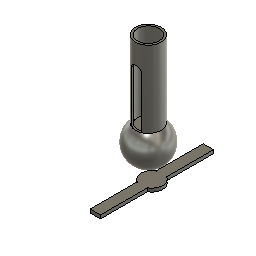
Tube and Handle (Autodesk Fusion 360 design; units mm, degrees)
part number: 2026-07-05-17-09-31-092
Autodesk Fusion 360 part; units mm, degrees
sphere "SpherePrimitive1" add diameter 80 placed x (1, 0, 0) y (0, 0, -1) z (0, 1, 0) at (0, 0, 0) makes body 1
sketch "Sketch2" plane through (0, 0, 0) normal (0, 1, 0) x (1, 0, 0)
  circle A0 centre (0, 0) radius 25
  dimension "d2" = 50
  constraint coincident A0.centre origin
  measures "d2" diameter of A0
extrude "Extrude1" add sketch "Sketch2" along normal blind 200 bodies 1
hole "Hole1" at (0, 200, 0) direction (0, -1, 0) diameter 42 depth 170 tip angle 180 bodies 1
extrude "Extrude2" cut 1 faces at (23.554, 200, 1.7651) along direction (0, -1, 0) blind 20 on bodies 1 bodies 1
sketch "Sketch3" plane through (0, 0, 0) normal (0, 0, 1) x (1, 0, 0)
  line L0 (-25, 31.225) -> (25, 31.225)
  line L1 (-25, 180) -> (25, 180)
  line L2 (10, 31.225) -> (-10, 31.225)
  line L3 (-10, 31.225) -> (-10, 131.225)
  line L4 (10, 131.225) -> (10, 31.225)
  arc A0 (0, 141.225) -> (-10, 131.225) centre (0, 131.225) ccw
  arc A1 (10, 131.225) -> (0, 141.225) centre (0, 131.225) ccw
  point P0 (10, 141.225)
  dimension "d10" = 20
  dimension "d11" = 110
  dimension "d12" = 15
  dimension "d13" = 10
  dimension "d14" = 10
  constraint horizontal L2
  constraint vertical L3
  constraint vertical L4
  constraint coincident L0 L2.start
  constraint tangent L3 A0
  constraint coincident P0 L4
  constraint tangent L4 A1
  constraint coincident A0.start A1.end
  measures "d10" distance of L2.start L2.end
  measures "d11" distance of L2.start P0
  measures "d12" distance of L0.end L4
  measures "d13" radius of A0
  measures "d14" radius of A1
extrude "Extrude3" cut sketch "Sketch3" along normal blind 30 and the other way blind 50 bodies 1
sketch "Sketch4" plane through (0, 0, 0) normal (0, 1, 0) x (1, 0, 0)
  circle A0 centre (73.8522, -67.0113) radius 21
  line L0 (63.8522, 42.9887) -> (83.8522, 42.9887)
  line L1 (83.8522, 42.9887) -> (83.8522, -177.0113)
  line L2 (83.8522, -177.0113) -> (63.8522, -177.0113)
  line L3 (63.8522, -177.0113) -> (63.8522, 42.9887)
  dimension "d19" = 42
  dimension "d20" = 20
  dimension "d21" = 220
  dimension "d22" = 10
  dimension "d23" = 110
  constraint horizontal L0
  constraint vertical L1
  constraint horizontal L2
  constraint vertical L3
  measures "d19" diameter of A0
  measures "d20" distance of L0.start L0.end
  measures "d21" distance of L0.start L2.end
  measures "d22" distance of A0.centre L1
  measures "d23" distance of A0.centre L2
extrude "Extrude4" add sketch "Sketch4" along normal blind 6.7 separate body makes body 2
